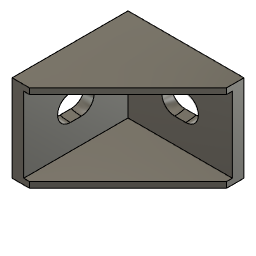
Small+90+Degree+Angle+Bracket (Autodesk Fusion 360 design; units mm, degrees)
Autodesk Fusion 360 part; units mm, degrees
sketch "Sketch1" plane through (0, 0, 0) normal (0, 1, 0) x (1, 0, 0)
  line L0 (0, 0) -> (20, 0)
  line L1 (0, -20) -> (0, 0)
  line L2 (20, 0) -> (20, -3)
  line L3 (0, -20) -> (3, -20)
  line L4 (3, -20) -> (20, -3)
  constraint horizontal L0
  constraint vertical L1
  constraint coincident L0.start L1.end
  constraint perpendicular L1 L3
extrude "Extrude1" add sketch "Sketch1" along normal blind 15
sketch "Sketch2" plane through (0, 0, 20) normal (0, 0, 1) x (1, 0, 0)
  line L0 (0, 0) -> (3, 0)
  line L1 (3, 0) -> (3, 15)
  line L2 (3, 15) -> (0, 15)
  line L3 (0, 15) -> (0, 0)
  line L4 (2, 14) -> (20, 14)
  line L5 (20, 14) -> (20, 1)
  line L6 (20, 1) -> (2, 1)
  line L7 (2, 1) -> (2, 14)
  constraint horizontal L4
  constraint vertical L5
  constraint horizontal L6
  constraint vertical L7
extrude "Extrude2" cut sketch "Sketch2" against normal blind 18 contours L1 L4 L6 L7 | L1 L4 L5 L6
sketch "Sketch3" plane through (0, 0, 2) normal (0, 0, 1) x (1, 0, 0)
  line L0 (2, 1) -> (20, 1)
  line L1 (20, 1) -> (20, 14)
  line L2 (20, 14) -> (2, 14)
  line L3 (2, 14) -> (2, 1)
  arc A0 (10.0508, 9.7) -> (10.0508, 5.3) centre (10.05, 7.5) ccw
  arc A1 (11.95, 5.3) -> (11.95, 9.7) centre (11.95, 7.5) ccw
  line L4 (10.0508, 9.7) -> (11.95, 9.7)
  line L5 (10.0508, 5.3) -> (11.95, 5.3)
  dimension "d5" = 4.4
  dimension "d6" = 4.4
  dimension "d8" = 1.9
  dimension "d9" = 8.05
  constraint tangent A1 L4
  constraint tangent A1 L5
  measures "d5" diameter of A0
  measures "d6" diameter of A1
  measures "d8" distance of A0.centre A1.centre
  measures "d9" distance of L1 A1.centre
revolve "Revolve1" cut sketch "Sketch3" angle 360 about axis through (2, 14, 2) along (0, -1, 0) contours A0 A1 L4 L5
equation "d8 = 6.3 mm - 4.4 mm"
